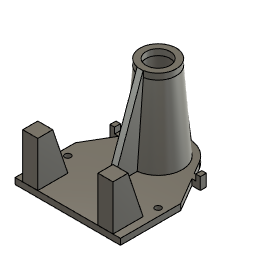
Pencil Mount V2 v4 (Autodesk Fusion 360 design; units mm, degrees)
Autodesk Fusion 360 part; units mm, degrees
note: some values were not read from the file. Set by a fixed rule: which sketch regions a step uses.
sketch "Sketch1" plane through (0, 0, 0) normal (1, 0, 0) x (0, 0, -1)
  line L0 (0, 0) -> (-4, 0)
  line L1 (-4, 0) -> (-4, 30)
  line L2 (-4, 30) -> (0, 30)
  line L3 (0, 30) -> (0, 0)
  line L4 (-4, 30) -> (-8, 30)
  line L5 (-8, 30) -> (-8, 0)
  line L6 (-8, 0) -> (-4, 0)
  line L7 (-4, 0) -> (-4, 30)
  line L8 (-4, 30) -> (-6, 30)
  line L9 (-6, 30) -> (-6, 28)
  line L10 (-6, 28) -> (-4, 28)
  line L11 (-4, 28) -> (-4, 30)
  line L12 (-4, 0) -> (-8, 0)
  line L13 (-8, 0) -> (-8, 2)
  line L14 (-8, 2) -> (-4, 2)
  line L15 (-4, 2) -> (-4, 0)
  line L16 (-6, 28) -> (-8, 2)
  spline S0 degree 5 poles (-4, 2) (-4.0818, 2.52) (-4.2384, 3.56) (-4.4517, 5.12) (-4.6926, 7.2) (-4.9161, 9.8) (-5.0551, 12.4) (-5.1027, 15) (-5.0551, 17.6) (-4.9161, 20.2) (-4.6926, 22.8) (-4.4517, 24.88) (-4.2384, 26.44) (-4.0818, 27.48) (-4, 28) knots 0 0 0 0 0 0 0.1 0.2 0.3 0.4 0.5 0.6 0.7 0.8 0.9 1 1 1 1 1 1
  point P0 (-5.079, 15)
  dimension "d1" = 4
  dimension "d2" = 30
  dimension "d3" = 4
  dimension "d4" = 30
  dimension "d5" = 2
  dimension "d6" = 2
  dimension "d7" = 2
  constraint horizontal L0
  constraint vertical L1
  constraint horizontal L2
  constraint vertical L3
  constraint coincident L0.start L3.end
  constraint horizontal L4
  constraint vertical L5
  constraint horizontal L6
  constraint vertical L7
  constraint horizontal L8
  constraint vertical L9
  constraint horizontal L10
  constraint vertical L11
  constraint horizontal L12
  constraint vertical L13
  constraint horizontal L14
  constraint vertical L15
  measures "d1" distance of L0.start L0.end
  measures "d2" distance of L0.start L2.end
  measures "d3" distance of L1.end L4.end
  measures "d4" distance of L1.end L0.end
  measures "d5" distance of L1.end L8.end
  measures "d6" distance of L1.end L10.end
  measures "d7" distance of L0.end L14.end
revolve "Revolve1" add sketch "Sketch1" angle 360 about axis through (0, 30, 0) along (0, -1, 0) contours L1 L5 L6 L7 L12 L13 L14 L15 | L10 L14 L16 S0 | L1 L4 L7 L8 L9 L10 L11
sketch "Sketch2" plane through (0, 0, 0) normal (0, -1, 0) x (1, 0, 0)
  circle A0 centre (0, 0) radius 4
  circle A1 centre (0, 0) radius 8
  line L0 (0, 0) -> (10, 0)
  line L1 (10, 0) -> (10, 10)
  line L2 (10, 10) -> (0, 10)
  line L3 (0, 10) -> (0, 0)
  line L4 (0, 0) -> (-10, 0)
  line L5 (-10, 0) -> (-10, 10)
  line L6 (-10, 10) -> (0, 10)
  line L7 (0, 10) -> (0, 0)
  line L8 (0, 0) -> (-10, 0)
  line L9 (-10, 0) -> (-10, -10)
  line L10 (-10, -10) -> (0, -10)
  line L11 (0, -10) -> (0, 0)
  line L12 (0, 0) -> (10, 0)
  line L13 (10, 0) -> (10, -10)
  line L14 (10, -10) -> (0, -10)
  line L15 (0, -10) -> (0, 0)
  line L16 (0, 15) -> (-15, 15)
  line L17 (-15, 15) -> (0, 15)
  line L18 (0, 15) -> (15, 15)
  line L19 (-17.5, 17.5) -> (17.5, 17.5)
  line L20 (17.5, 17.5) -> (17.5, 10)
  line L21 (17.5, 10) -> (-17.5, 10)
  line L22 (-17.5, 10) -> (-17.5, 17.5)
  circle A2 centre (-15, 15) radius 1
  circle A3 centre (15, 15) radius 1
  line L23 (-10, -8) -> (10, -8)
  circle A4 centre (0, 0) radius 10
  dimension "d9" = 15
  dimension "d10" = 15
  dimension "d11" = 2
  dimension "d12" = 2
  constraint horizontal L0
  constraint vertical L1
  constraint horizontal L2
  constraint vertical L3
  constraint coincident A0.centre A1.centre
  constraint horizontal L4
  constraint vertical L5
  constraint horizontal L6
  constraint vertical L7
  constraint horizontal L8
  constraint vertical L9
  constraint horizontal L10
  constraint vertical L11
  constraint horizontal L12
  constraint vertical L13
  constraint horizontal L14
  constraint vertical L15
  constraint horizontal L16
  constraint parallel L16 L17
  constraint parallel L17 L18
  constraint horizontal L19
  constraint vertical L20
  constraint horizontal L21
  constraint vertical L22
  constraint coincident L16.end L17.start
  constraint coincident L9 L23.start
  constraint coincident L13 L23.end
  constraint perpendicular L13 L23
  constraint coincident L4.end A4
  measures "d9" distance of L16.start L16.end
  measures "d10" distance of L16.start L18.end
  measures "d11" diameter of A2
  measures "d12" diameter of A3
extrude "Extrude1" add sketch "Sketch2" against normal blind 2 contours A1 L0 L12 L23 A4 | A1 L0 L3 L7 L12 A4 | A1 L3 L4 L7 L8 A4 | A1 L4 L8 L23 A4 | L11 L15 L23 A4 | L11 L15 L23 A4 | L1 L2 L21 A4 | L2 L6 L19 L20 L21 L22 | L5 L6 L21 A4
sketch "Sketch3" plane through (0, 0, 0) normal (1, 0, 0) x (0, 0, -1)
  line L0 (-6, 30) -> (-16, 2)
  line L1 (-16, 2) -> (-7, 2)
  line L2 (-7, 2) -> (-5, 28)
  line L3 (-5, 28) -> (-5, 30)
  line L4 (-5, 30) -> (-6, 30)
  constraint horizontal L1
  constraint perpendicular L1 L3
  constraint perpendicular L3 L4
extrude "Extrude2" add sketch "Sketch3" along normal mid plane 2
sketch "Sketch4" plane through (0, 0, 0) normal (1, 0, 0) x (0, 0, -1)
  line L0 (6, 30) -> (10, 2)
  line L1 (10, 2) -> (7, 2)
  line L2 (7, 2) -> (5, 28)
  line L3 (5, 28) -> (5, 30)
  line L4 (5, 30) -> (6, 30)
  constraint horizontal L1
  constraint vertical L3
  constraint parallel L1 L4
extrude "Extrude3" add sketch "Sketch4" along normal mid plane 2
sketch "Sketch5" plane through (0, 0, 0) normal (0, -1, 0) x (1, 0, 0)
  arc A0 (-10, 0) -> (10, 0) centre (0, 0) ccw
  line L0 (10, 0) -> (10, 10)
  line L1 (10, 10) -> (17.5, 10)
  line L2 (17.5, 10) -> (17.5, 17.5)
  line L3 (17.5, 17.5) -> (-17.5, 17.5)
  line L4 (-17.5, 17.5) -> (-17.5, 10)
  line L5 (-17.5, 10) -> (-10, 10)
  line L6 (-10, 10) -> (-10, 0)
  circle A1 centre (15, 15) radius 1
  circle A2 centre (-15, 15) radius 1
  circle A3 centre (0, 0) radius 4
  line L7 (-17.5, 10) -> (-8.6154, -5.0769)
  line L8 (17.5, 10) -> (8.6154, -5.0769)
  constraint coincident L4.end L5.start
  constraint coincident A0 L7.end
  constraint tangent A0 L7
  constraint coincident L1.end L2.start
  constraint coincident A0 L8.end
  constraint tangent A0 L8
extrude "Extrude4" add sketch "Sketch5" against normal blind 2 contours A0 L5 L6 L7 | A0 L0 L1 L8
sketch "Sketch6" plane through (0, 0, 0) normal (0, -1, 0) x (1, 0, 0)
  arc A0 (-8.6154, -5.0769) -> (8.6154, -5.0769) centre (0, 0) ccw
  line L0 (8.6154, -5.0769) -> (17.5, 10)
  line L1 (17.5, 10) -> (17.5, 17.5)
  line L2 (17.5, 17.5) -> (-17.5, 17.5)
  line L3 (-17.5, 17.5) -> (-17.5, 10)
  line L4 (-17.5, 10) -> (-8.6154, -5.0769)
  circle A1 centre (15, 15) radius 1
  circle A2 centre (-15, 15) radius 1
  circle A3 centre (0, 0) radius 4
  line L5 (10, -1) -> (15, -1)
  line L6 (15, -1) -> (15, 1)
  line L7 (15, 1) -> (10, 1)
  line L8 (10, 1) -> (10, -1)
  line L9 (-10, -1) -> (-15, -1)
  line L10 (-15, -1) -> (-15, 1)
  line L11 (-15, 1) -> (-10, 1)
  line L12 (-10, 1) -> (-10, -1)
  constraint horizontal L5
  constraint vertical L6
  constraint horizontal L7
  constraint vertical L8
  constraint horizontal L9
  constraint vertical L10
  constraint horizontal L11
  constraint vertical L12
extrude "Extrude5" add sketch "Sketch6" against normal blind 2 contours L4 L9 L10 L11 | L0 L5 L6 L7
sketch "Sketch7" plane through (0, 2, 0) normal (0, 1, 0) x (-1, 0, 0)
  line L0 (1, -7.9373) -> (1, -9.9499)
  arc A0 (1, -9.9499) -> (8.6154, -5.0769) centre (0, 0) ccw
  line L1 (8.6154, -5.0769) -> (11.0179, -1)
  line L2 (11.0179, -1) -> (15, -1)
  line L3 (15, -1) -> (15, 1)
  line L4 (15, 1) -> (12.1964, 1)
  line L5 (12.1964, 1) -> (17.5, 10)
  line L6 (17.5, 10) -> (17.5, 17.5)
  line L7 (17.5, 17.5) -> (-17.5, 17.5)
  line L8 (-17.5, 17.5) -> (-17.5, 10)
  line L9 (-17.5, 10) -> (-12.1964, 1)
  line L10 (-12.1964, 1) -> (-15, 1)
  line L11 (-15, 1) -> (-15, -1)
  line L12 (-15, -1) -> (-11.0179, -1)
  line L13 (-11.0179, -1) -> (-8.6154, -5.0769)
  arc A1 (-8.6154, -5.0769) -> (-1, -9.9499) centre (0, 0) ccw
  line L14 (-1, -9.9499) -> (-1, -7.9373)
  arc A2 (-1, 7.9373) -> (-1, -7.9373) centre (0, 0) ccw
  line L15 (-1, 7.9373) -> (-1, 16)
  line L16 (-1, 16) -> (1, 16)
  line L17 (1, 16) -> (1, 7.9373)
  arc A3 (1, -7.9373) -> (1, 7.9373) centre (0, 0) ccw
  circle A4 centre (15, 15) radius 1
  circle A5 centre (-15, 15) radius 1
  line L18 (15, -1) -> (13.5, -1)
  line L19 (13.5, -1) -> (13.5, 1)
  line L20 (13.5, 1) -> (15, 1)
  line L21 (15, 1) -> (15, -1)
  line L22 (-15, -1) -> (-13.5, -1)
  line L23 (-13.5, -1) -> (-13.5, 1)
  line L24 (-13.5, 1) -> (-15, 1)
  line L25 (-15, 1) -> (-15, -1)
  dimension "d23" = 1.5
  dimension "d24" = 1.5
  constraint horizontal L18
  constraint vertical L19
  constraint horizontal L20
  constraint vertical L21
  constraint coincident L2.end L3.start
  constraint horizontal L22
  constraint vertical L23
  constraint horizontal L24
  constraint vertical L25
  constraint coincident L11.end L12.start
  measures "d23" distance of L2.end L18.end
  measures "d24" distance of L11.end L22.end
extrude "Extrude6" add sketch "Sketch7" along normal blind 2 contours L2 L3 L4 L18 L19 L20 L21 | L10 L11 L12 L22 L23 L24 L25
sketch "Sketch8" plane through (0, 0, 0) normal (0, -1, 0) x (1, 0, 0)
  arc A0 (-8.6154, -5.0769) -> (8.6154, -5.0769) centre (0, 0) ccw
  line L0 (8.6154, -5.0769) -> (11.0179, -1)
  line L1 (11.0179, -1) -> (15, -1)
  line L2 (15, -1) -> (15, 1)
  line L3 (15, 1) -> (12.1964, 1)
  line L4 (12.1964, 1) -> (17.5, 10)
  line L5 (17.5, 10) -> (17.5, 17.5)
  line L6 (17.5, 17.5) -> (-17.5, 17.5)
  line L7 (-17.5, 17.5) -> (-17.5, 10)
  line L8 (-17.5, 10) -> (-12.1964, 1)
  line L9 (-12.1964, 1) -> (-15, 1)
  line L10 (-15, 1) -> (-15, -1)
  line L11 (-15, -1) -> (-11.0179, -1)
  line L12 (-11.0179, -1) -> (-8.6154, -5.0769)
  circle A1 centre (15, 15) radius 1
  circle A2 centre (-15, 15) radius 1
  circle A3 centre (0, 0) radius 4
  line L13 (-17.5, 15.0174) -> (17.5, 15.0174)
  line L14 (17.5, 15.0174) -> (17.5, 30.0174)
  line L15 (17.5, 30.0174) -> (-17.5, 30.0174)
  line L16 (-17.5, 30.0174) -> (-17.5, 15.0174)
  dimension "d27" = 35
  dimension "d28" = 15
  constraint horizontal L13
  constraint vertical L14
  constraint horizontal L15
  constraint vertical L16
  constraint coincident L7 L13.start
  measures "d27" distance of L13.start L13.end
  measures "d28" distance of L13.start L15.end
extrude "Extrude7" add sketch "Sketch8" against normal blind 2 contours L6 L14 L15 L16
sketch "Sketch9" plane through (0, 2, 0) normal (0, 1, 0) x (-1, 0, 0)
  circle A0 centre (-15, 15) radius 1
  circle A1 centre (15, 15) radius 1
  line L0 (13.5, -1) -> (13.5, 1)
  line L1 (13.5, 1) -> (12.1964, 1)
  line L2 (12.1964, 1) -> (17.5, 10)
  line L3 (17.5, 10) -> (17.5, 30.0174)
  line L4 (17.5, 30.0174) -> (-17.5, 30.0174)
  line L5 (-17.5, 30.0174) -> (-17.5, 10)
  line L6 (-17.5, 10) -> (-12.1964, 1)
  line L7 (-12.1964, 1) -> (-13.5, 1)
  line L8 (-13.5, 1) -> (-13.5, -1)
  line L9 (-13.5, -1) -> (-11.0179, -1)
  line L10 (-11.0179, -1) -> (-8.6154, -5.0769)
  arc A2 (-8.6154, -5.0769) -> (-1, -9.9499) centre (0, 0) ccw
  line L11 (-1, -9.9499) -> (-1, -7.9373)
  arc A3 (-1, 7.9373) -> (-1, -7.9373) centre (0, 0) ccw
  line L12 (-1, 7.9373) -> (-1, 16)
  line L13 (-1, 16) -> (1, 16)
  line L14 (1, 16) -> (1, 7.9373)
  arc A4 (1, -7.9373) -> (1, 7.9373) centre (0, 0) ccw
  line L15 (1, -7.9373) -> (1, -9.9499)
  arc A5 (1, -9.9499) -> (8.6154, -5.0769) centre (0, 0) ccw
  line L16 (8.6154, -5.0769) -> (11.0179, -1)
  line L17 (11.0179, -1) -> (13.5, -1)
  line L18 (15, 25) -> (10, 25)
  line L19 (10, 25) -> (10, 30)
  line L20 (10, 30) -> (15, 30)
  line L21 (15, 30) -> (15, 25)
  line L22 (-15, 25) -> (-10, 25)
  line L23 (-10, 25) -> (-10, 30)
  line L24 (-10, 30) -> (-15, 30)
  line L25 (-15, 30) -> (-15, 25)
  line L26 (-10, 25) -> (-1, 7.9373)
  line L27 (-15, 25) -> (-5.0752, 6.184)
  line L28 (10, 25) -> (1, 7.9373)
  line L29 (15, 25) -> (5.0752, 6.184)
  dimension "d31" = 5
  dimension "d32" = 5
  constraint horizontal L18
  constraint vertical L19
  constraint horizontal L20
  constraint vertical L21
  constraint horizontal L22
  constraint vertical L23
  constraint horizontal L24
  constraint vertical L25
  constraint coincident A3.start L12.start
  constraint coincident A3 L27.end
  constraint parallel L26 L27
  constraint coincident L14.end A4.end
  constraint coincident A4 L29.end
  constraint parallel L28 L29
  measures "d31" distance of L18.start L18.end
  measures "d32" distance of L18.start L20.end
extrude "Extrude8" add sketch "Sketch9" along normal blind 15 contours L18 L19 L20 L21 | L22 L23 L24 L25
sketch "Sketch10" plane through (15, 0, 0) normal (1, 0, 0) x (0, 0, -1)
  line L0 (-30, 2) -> (-25, 2)
  line L1 (-25, 2) -> (-25, 17)
  line L2 (-25, 17) -> (-30, 17)
  line L3 (-30, 17) -> (-30, 2)
  line L4 (-25, 17) -> (-20, 17)
  line L5 (-20, 17) -> (-20, 2)
  line L6 (-20, 2) -> (-25, 2)
  line L7 (-25, 2) -> (-25, 17)
  line L8 (-25, 17) -> (-20, 2)
  constraint horizontal L4
  constraint vertical L5
  constraint horizontal L6
  constraint vertical L7
  constraint coincident L1.end L2.start
extrude "Extrude9" add sketch "Sketch10" against normal blind 5 contours L1 L6 L7 L8
sketch "Sketch11" plane through (-15, 0, 0) normal (-1, 0, 0) x (0, 0, 1)
  line L0 (25, 2) -> (30, 2)
  line L1 (30, 2) -> (30, 17)
  line L2 (30, 17) -> (25, 17)
  line L3 (25, 17) -> (25, 2)
  line L4 (25, 17) -> (20, 17)
  line L5 (20, 17) -> (20, 2)
  line L6 (20, 2) -> (25, 2)
  line L7 (25, 2) -> (25, 17)
  line L8 (25, 17) -> (20, 2)
  constraint horizontal L4
  constraint vertical L5
  constraint horizontal L6
  constraint vertical L7
  constraint coincident L2.end L3.start
extrude "Extrude10" add sketch "Sketch11" against normal blind 5 contours L3 L6 L7 L8
